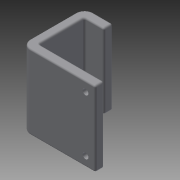
# Autodesk Inventor part: GUS SHOULDER MOUNT
Saved by Autodesk Inventor 2013 (Build 170138000, 138)
## iProperties
Created: 2014-01-03
Part Number: GUS SHOULDER MOUNT
Material: Generic
Document SubType Name: Modeling
Designer: employee
Density: 1 g/cm^3
Author: employee
Autodesk Inventor part; units mm, degrees
ref_plane "YZ Plane" through (0, 0, 0) normal (1, 0, 0) x (0, 1, 0)
ref_plane "XZ Plane" through (0, 0, 0) normal (0, 1, 0) x (-1, 0, 0)
ref_plane "XY Plane" through (0, 0, 0) normal (0, 0, 1) x (1, 0, 0)
sketch "Sketch1" plane through (0, 0, 0) normal (0, 0, 1) x (1, 0, 0)
  line L0 (41.4, 0) -> (0, 0)
  line L1 (0, 0) -> (0, 35.4)
  line L2 (0, 35.4) -> (15.8314, 35.4)
  line L3 (15.8314, 35.4) -> (15.8314, 30.4)
  line L4 (15.8314, 30.4) -> (5, 30.4)
  line L5 (5, 30.4) -> (5, 5)
  line L6 (5, 5) -> (41.4, 5)
  line L7 (41.4, 5) -> (41.4, 0)
  dimension "d0" = 5
  dimension "d2" = 5
  dimension "d3" = 25.4
  dimension "d4" = 36.4
  constraints: 16 end point, 7 parallel, 1 horizontal, 1 perpendicular
  measures "d0" distance of L6.end L0.start
  measures "d2" distance between parallel lines of L1 L5
  measures "d3" distance of L4.end L5.end
  measures "d4" distance of L5.end L6.end
extrude "Extrusion1" add sketch "Sketch1" along normal blind 42
fillet "Fillet1" radius 5 2 edges at (0, 35.4, 21) (0, 0, 21)
fillet "Fillet2" radius 1 2 edges at (5, 5, 21) (5, 30.4, 21)
sketch "Sketch2" plane through (41.4, 0, 0) normal (0, -1, 0) x (1, 0, 0)
  line L0 (0, 0) -> (0, 42) projected
  line L1 (-36.4, 42) -> (0, 42) projected
  line L2 (-5.5, 36.5) -> (-5.5, 5.5)
  circle A0 centre (-5.5, 36.5) radius 1.6
  circle A1 centre (-5.5, 5.5) radius 1.6
  point P0 (-41.4, 0)
  point P1 (-5.5, 21)
  point P2 (0, 21)
  dimension "d9" = 31
  dimension "d11" = 35.9
  dimension "d12" = 3.2
  dimension "d13" = 3.2
  constraints: 2 centre point, 2 coincident, 2 end point, 2 midpoint, 1 horizontal alignment, 1 perpendicular
  measures "d9" distance of L2.start L2.end
  measures "d11" distance from line of L2 point (-41.4, 0)
  measures "d12" diameter of A0
  measures "d13" diameter of A1
extrude "Extrusion2" cut sketch "Sketch2" against normal through all
fillet "Fillet3" radius 1 28 edges at (1.4645, 1.4645, 42) (23.2, 0, 42) (41.4, 2.5, 42) (23.7, 5, 42) (5.2929, 5.2929, 42) (5, 17.7, 42) (5.2929, 30.1071, 42) (10.9157, 30.4, 42) (15.8314, 32.9, 42) (10.4157, 35.4, 42) (1.4645, 33.9355, 42) (0, 17.7, 42) (1.4645, 1.4645, 0) (0, 17.7, 0) (1.4645, 33.9355, 0) (10.4157, 35.4, 0) (15.8314, 32.9, 0) (10.9157, 30.4, 0) (5.2929, 30.1071, 0) (5, 17.7, 0) (5.2929, 5.2929, 0) (23.7, 5, 0) (41.4, 2.5, 0) (23.2, 0, 0) (41.4, 5, 21) (41.4, 0, 21) (15.8314, 35.4, 21) (15.8314, 30.4, 21)
body "Solid1"
